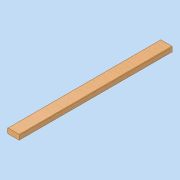
# Autodesk Inventor part: 2x4
Saved by Autodesk Inventor 2019 (Build 230136000, 136)
## iProperties
Created: 2019-12-05
Part Number: 2x4
Material: Pine
Document SubType Name: Modeling
Designer: qitilab4
Density: 0.570257 g/cm^3
Appearance: Yellow Pine - Solid Natural Low Gloss
Author: qitilab4
Autodesk Inventor part; units mm, degrees
ref_plane "YZ Plane" through (0, 0, 0) normal (1, 0, 0) x (0, 1, 0)
ref_plane "XZ Plane" through (0, 0, 0) normal (0, 1, 0) x (-1, 0, 0)
ref_plane "XY Plane" through (0, 0, 0) normal (0, 0, 1) x (1, 0, 0)
sketch "Sketch1" plane through (0, 0, 0) normal (0, 1, 0) x (-1, 0, 0)
  line L0 (44.45, -571.5) -> (-44.45, -571.5)
  line L1 (-44.45, -571.5) -> (-44.45, 571.5)
  line L2 (-44.45, 571.5) -> (44.45, 571.5)
  line L3 (44.45, 571.5) -> (44.45, -571.5)
  line L4 (44.45, -571.5) -> (-44.45, 571.5) construction
  line L5 (-44.45, -571.5) -> (44.45, 571.5) construction
  point P0 (0, 0)
  dimension "d0" = 88.9
  dimension "d1" = 1143
  constraints: 12 end point, 2 midpoint, 2 parallel, 1 horizontal, 1 perpendicular
  measures "d0" distance of L1.end L2.end
  measures "d1" distance of L0.end L1.end
extrude "Extrusion1" add sketch "Sketch1" along normal blind 38.1
fillet "Fillet1" radius 3.175 4 edges at (44.45, 38.1, 0) (44.45, 0, 0) (-44.45, 38.1, 0) (-44.45, 0, 0)
body "Solid1"
